led_strip_holder (Autodesk Fusion 360 design; units mm, degrees)
Autodesk Fusion 360 part; units mm, degrees
sketch "Sketch1" plane through (0, 0, 0) normal (0, 1, 0) x (1, 0, 0)
  line L0 (-24.5, 0) -> (-24.5, -2)
  line L1 (-24.5, -2) -> (-19.5, -2)
  line L2 (-19.5, -2) -> (-19.5, -4.5)
  line L3 (-19.5, -4.5) -> (-5, -4.5)
  line L4 (-5, -4.5) -> (-5, -2)
  line L5 (-5, -2) -> (0, -2)
  line L6 (0, -2) -> (0, 0)
  line L7 (-24.5, 0) -> (-17.5, 0)
  line L8 (-17.5, 0) -> (-17.5, -3)
  line L9 (-17.5, -3) -> (-7, -3)
  line L10 (-7, -3) -> (-7, 0)
  line L11 (-7, 0) -> (0, 0)
  dimension "d1" = 10.5
  dimension "d3" = 2
  dimension "d4" = 2
  dimension "d8" = 7
  dimension "d9" = 7
  dimension "d10" = 2
  dimension "d13" = 2
  dimension "d14" = 3
  dimension "d15" = 2.5
  constraint vertical L0
  constraint perpendicular L0 L1
  constraint perpendicular L1 L2
  constraint perpendicular L0 L3
  constraint perpendicular L1 L4
  constraint perpendicular L4 L5
  constraint perpendicular L5 L6
  constraint perpendicular L0 L7
  constraint perpendicular L7 L8
  constraint perpendicular L0 L9
  constraint perpendicular L9 L10
  constraint perpendicular L6 L11
  constraint coincident L6.end L11.end
  constraint collinear L7 L11
  measures "d1" distance of L8.end L9.end
  measures "d3" distance of L2 L8
  measures "d4" distance of L4 L10
  measures "d8" distance of L6.end L10.end
  measures "d9" distance of L0.start L7.end
  measures "d10" distance of L0.start L0.end
  measures "d13" distance of L5.end L6.end
  measures "d14" distance of L9.end L10.end
  measures "d15" distance of L3.end L4.end
extrude "Extrude1" add sketch "Sketch1" along normal blind 104.5
sketch "Sketch3" plane through (0, 0, 4.5) normal (0, 0, 1) x (-1, 0, 0)
  line L0 (19.5, 0) -> (5, 0)
  line L1 (5, 0) -> (5, -104.5)
  line L2 (5, -104.5) -> (19.5, -104.5)
  line L3 (19.5, -104.5) -> (19.5, 0)
  line L4 (24.5, -10) -> (0, -10)
  line L5 (0, -10) -> (0, -10.5)
  line L6 (0, -10.5) -> (24.5, -10.5)
  line L7 (24.5, -10.5) -> (24.5, -10)
  dimension "d25" = 0.5
  dimension "d26" = 10
  dimension "d27" = 5
  dimension "d28" = 5
  constraint horizontal L4
  constraint vertical L5
  constraint horizontal L6
  constraint vertical L7
  measures "d25" distance of L4.start L6.end
  measures "d26" distance of L0 L4
  measures "d27" distance of L3 L6.end
  measures "d28" distance of L1.end L5
extrude "Extrude2" cut sketch "Sketch3" against normal blind 3.8 contours L3 L4 L6 L7 | L1 L3 L4 L6 | L1 L4 L5 L6
pattern_path "PathPattern1" count 9 spacing 10.5 from (-5, 10.5, 4.5) along 1 edges at (-5, 57.5, 4.5) of "Extrude2"
